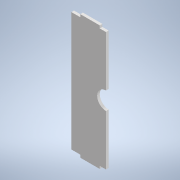
# Autodesk Inventor part: ACHTERKANT
Saved by Autodesk Inventor 2021 (Build 250183000, 183)
## iProperties
Created: 2022-02-02
Part Number: ACHTERKANT
Material: Generic
Document SubType Name: Modeling
Designer: ryan
Density: 1 g/cm^3
Appearance: Default
Author: ryan
Autodesk Inventor part; units mm, degrees
ref_plane "YZ Plane" through (0, 0, 0) normal (1, 0, 0) x (0, 1, 0)
ref_plane "XZ Plane" through (0, 0, 0) normal (0, 1, 0) x (-1, 0, 0)
ref_plane "XY Plane" through (0, 0, 0) normal (0, 0, 1) x (1, 0, 0)
sketch "Sketch1" plane through (0, 0, 0) normal (0, 0, 1) x (1, 0, 0)
  line L0 (0, 0) -> (0, -3)
  line L1 (0, -3) -> (7, -3)
  line L2 (7, -3) -> (7, 0)
  line L3 (0, 0) -> (-22, 0)
  line L4 (-22, 0) -> (-22, -3)
  line L5 (-22, -3) -> (0, -3)
  line L6 (0, -3) -> (0, 0)
  line L7 (-22, 0) -> (-32, 0)
  line L8 (-32, 0) -> (-32, -3)
  line L9 (-32, -3) -> (-22, -3)
  line L10 (-22, -3) -> (-22, 0)
  line L11 (-32, 0) -> (7, 0)
  line L12 (7, 0) -> (7, -70)
  line L13 (7, -70) -> (-32, -70)
  line L14 (-32, -70) -> (-32, 0)
  circle A0 centre (7, -70) radius 10
  point P0 (-3, -70)
  point P1 (7, -60)
  dimension "d0" = 3
  dimension "d1" = 7
  dimension "d2" = 22
  dimension "d3" = 3
  dimension "d4" = 10
  dimension "d5" = 3
  dimension "d6" = 39
  dimension "d7" = 70
  dimension "d8" = 20
  constraints: 30 end point, 6 parallel, 4 perpendicular, 3 horizontal, 2 vertical, 1 centre point, 1 coincident
  measures "d0" distance of L0.start L0.end
  measures "d1" distance of L0.end L1.end
  measures "d2" distance of L5.end L4.end
  measures "d3" distance of L4.end L3.end
  measures "d4" distance of L9.end L8.end
  measures "d5" distance of L8.end L7.end
  measures "d6" distance of L12.end L13.end
  measures "d7" distance of L11.end L12.end
  measures "d8" diameter of A0
extrude "Extrusion1" add sketch "Sketch1" along normal blind 3 contours L0 L5 L4 L3 | L1 L12 A0 L13 L14 L9 L5
mirror "Mirror1" about plane through (-32, -70, 0) normal (0, -1, 0) of "Extrusion1"
sketch "Sketch2" plane through (-32, -3, 0) normal (-1, 0, 0) x (0, 0, 1)
  line L0 (0, 0) -> (3, 0)
  line L1 (3, 0) -> (3, -17)
  line L2 (3, -17) -> (0, -17)
  line L3 (0, -17) -> (0, 0)
  line L4 (3, -17) -> (0, -17)
  line L5 (0, -17) -> (0, -37)
  line L6 (0, -37) -> (3, -37)
  line L7 (3, -37) -> (3, -17)
  line L8 (0, -37) -> (3, -37)
  line L9 (3, -37) -> (3, -57)
  line L10 (3, -57) -> (0, -57)
  line L11 (0, -57) -> (0, -37)
  point P0 (0, 3)
  dimension "d11" = 3
  dimension "d12" = 17
  dimension "d13" = 3
  dimension "d14" = 20
  dimension "d15" = 3
  dimension "d16" = 20
  constraints: 24 end point, 6 parallel, 3 horizontal, 3 perpendicular
  measures "d11" distance of L1.end L2.end
  measures "d12" distance of L0.end L1.end
  measures "d13" distance of L6.end L5.end
  measures "d14" distance of L5.end L4.end
  measures "d15" distance of L9.end L10.end
  measures "d16" distance of L8.end L9.end
extrude "Extrusion2" add sketch "Sketch2" along normal blind 3 contours L2 L7 L6 L5
sketch "Sketch3" plane through (-32, -137, 0) normal (-1, 0, 0) x (0, 0, 1)
  line L0 (0, 97) -> (3, 97)
  line L1 (3, 97) -> (3, 77)
  line L2 (3, 77) -> (0, 77)
  line L3 (0, 77) -> (0, 97)
  line L4 (3, 77) -> (0, 77)
  line L5 (0, 77) -> (0, 57)
  line L6 (0, 57) -> (3, 57)
  line L7 (3, 57) -> (3, 77)
  line L8 (0, 97) -> (0, 0) projected
  line L9 (3, 57) -> (0, 57)
  line L10 (0, 57) -> (0, 37)
  line L11 (0, 37) -> (3, 37)
  line L12 (3, 37) -> (3, 57)
  point P0 (0, 137)
  dimension "d19" = 3
  dimension "d20" = 20
  dimension "d21" = 3
  dimension "d22" = 20
  dimension "d23" = 20
  constraints: 24 end point, 6 parallel, 3 horizontal, 3 perpendicular, 1 point on line
  measures "d19" distance of L1.end L2.end
  measures "d20" distance of L0.end L1.end
  measures "d21" distance of L6.end L5.end
  measures "d22" distance of L5.end L4.end
  measures "d23" distance of L10.end L9.end
extrude "Extrusion3" add sketch "Sketch3" along normal blind 3 contours L2 L7 L6 L5
sketch "Sketch4" plane through (-32, -137, 0) normal (-1, 0, 0) x (0, 0, 1)
  line L0 (2.7004, 57) -> (3, 37.0022)
  line L1 (3, 57) -> (3, 0) projected
  line L2 (0, 57) -> (0, 0) projected
  line L3 (3, 37.0022) -> (0, 37.0022)
  line L4 (0, 37.0022) -> (0, 17.0022)
  line L5 (0, 17.0022) -> (3, 17.0022)
  line L6 (3, 17.0022) -> (3, 37.0022)
  point P0 (0, 137)
  point P1 (3, 17.0022)
  point P2 (0, 37.0022)
  dimension "d26" = 20
  dimension "d27" = 20
  constraints: 10 end point, 2 parallel, 2 point on line, 1 horizontal, 1 perpendicular
  measures "d26" distance of L0.start L0.end
  measures "d27" distance of L4.end L3.end
extrude "Extrusion4" add sketch "Sketch4" along normal blind 3
body "Solid1"
